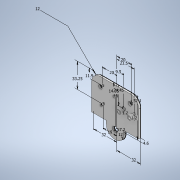
# Autodesk Inventor part: ENDER 3 E_PLATE
Saved by Autodesk Inventor 2022 (Build 260153070, 153G)
## iProperties
Created: 2022-01-01
Part Number: ENDER 3 E_PLATE
Material: Generic
Document SubType Name: Modeling
Designer: a laptop
Density: 1 g/cm^3
Appearance: Default
Author: a laptop
Autodesk Inventor part; units mm, degrees
ref_plane "YZ Plane" through (0, 0, 0) normal (1, 0, 0) x (0, 1, 0)
ref_plane "XZ Plane" through (0, 0, 0) normal (0, 1, 0) x (-1, 0, 0)
ref_plane "XY Plane" through (0, 0, 0) normal (0, 0, 1) x (1, 0, 0)
sketch "Sketch1" plane through (0, 0, 0) normal (0, 0, 1) x (1, 0, 0)
  circle A0 centre (0, 0) radius 3.6
  line L0 (32, 4.6) -> (12, 4.6)
  line L1 (-32, 4.6) -> (-32, 40.1)
  line L2 (-20, 52.1) -> (20, 52.1)
  line L3 (32, 40.1) -> (32, 4.6)
  circle A1 centre (-19, 18.85) radius 2
  circle A2 centre (-1.5, 37.75) radius 2
  circle A3 centre (9.5, 27.65) radius 1.5
  circle A4 centre (23.5, 27.65) radius 1.5
  circle A5 centre (9.5, 27.65) radius 2.7
  circle A6 centre (23.5, 27.65) radius 2.7
  circle A7 centre (-20, 40.2) radius 2.5
  circle A8 centre (-19, 18.85) radius 1.5
  circle A9 centre (-1.5, 37.75) radius 1.5
  circle A10 centre (20, 40.2) radius 2.5
  arc A11 (-20, 52.1) -> (-32, 40.1) centre (-20, 40.1) ccw
  arc A12 (32, 40.1) -> (20, 52.1) centre (20, 40.1) ccw
  arc A13 (-12, 0) -> (12, 0) centre (0, 0) ccw
  line L4 (-12, 0) -> (-12, 4.6)
  line L5 (12, 4.6) -> (12, 0)
  line L6 (-12, 4.6) -> (-32, 4.6)
  point P0 (-32, 52.1)
  dimension "d0" = 7.2
  dimension "d1" = 52.1
  dimension "d2" = 4.6
  dimension "d3" = 32
  dimension "d4" = 32
  dimension "d5" = 4
  dimension "d6" = 33.25
  dimension "d7" = 19
  dimension "d8" = 4
  dimension "d9" = 1.5
  dimension "d10" = 14.35
  dimension "d11" = 3
  dimension "d12" = 9.5
  dimension "d13" = 24.45
  dimension "d14" = 3
  dimension "d15" = 23.5
  dimension "d16" = 1.2
  dimension "d17" = 1.2
  dimension "d18" = 20
  dimension "d19" = 11.9
  dimension "d20" = 5
  dimension "d21" = 3
  dimension "d22" = 3
  dimension "d23" = 5
  dimension "d24" = 20
  dimension "d25" = 12
  dimension "d27" = 12
  constraints: 14 centre point, 14 end point, 6 point on circle, 6 tangent, 4 concentric, 4 parallel, 4 perpendicular, 3 point on line, 2 coincident, 2 horizontal, 2 horizontal alignment, 1 equal radius
  measures "d0" diameter of A0
  measures "d1" distance from line of L2 point (0, 0)
  measures "d2" distance from line of point (0, 0) L0
  measures "d3" distance from line of point (0, 0) L1
  measures "d4" distance from line of point (0, 0) L3
  measures "d5" diameter of A1
  measures "d6" vertical distance of point (-32, 52.1) A1.centre
  measures "d7" horizontal distance of point (0, 0) A1.centre
  measures "d8" diameter of A2
  measures "d9" horizontal distance of point (0, 0) A2.centre
  measures "d10" distance from line of L2 A2.centre
  measures "d11" diameter of A3
  measures "d12" horizontal distance of point (0, 0) A3.centre
  measures "d13" distance from line of L2 A3.centre
  measures "d14" diameter of A4
  measures "d15" horizontal distance of point (0, 0) A4.centre
  measures "d16" radial gap between concentric circles of A5 A3
  measures "d17" radial gap between concentric circles of A4 A6
  measures "d18" horizontal distance of point (0, 0) A7.centre
  measures "d19" vertical distance of point (-32, 52.1) A7.centre
  measures "d20" diameter of A7
  measures "d21" diameter of A8
  measures "d22" diameter of A9
  measures "d23" diameter of A10
  measures "d24" horizontal distance of point (0, 0) A10.centre
  measures "d25" radius of A11
  measures "d27" radius of A13
extrude "Extrusion1" add sketch "Sketch1" along normal blind 2.5 contours L0 L5 A13 L4 L6 L1 A11 L2 A12 L3
extrude "Extrusion2" add sketch "Sketch1" along normal blind 7 contours A5 | A6
extrude "Extrusion3" add sketch "Sketch1" along normal blind 2.5 and the other way blind 1.5 contours A1 | A2
body "Solid1"
